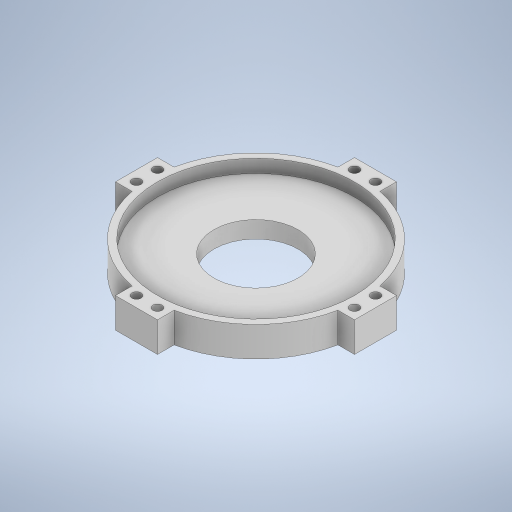
# Autodesk Inventor part: CO-0-01-PlanetaryCap
Saved by Autodesk Inventor 2023 (Build 270158000, 158)
## iProperties
Created: 2023-09-29
Part Number: CO-0-01-PlanetaryCap
Material: Generic
Document SubType Name: Modeling
Designer: thesl
Density: 1 g/cm^3
Appearance: Default
Author: thesl
Autodesk Inventor part; units mm, degrees
ref_plane "YZ Plane" through (0, 0, 0) normal (1, 0, 0) x (0, 1, 0)
ref_plane "XZ Plane" through (0, 0, 0) normal (0, 1, 0) x (-1, 0, 0)
ref_plane "XY Plane" through (0, 0, 0) normal (0, 0, 1) x (1, 0, 0)
sketch "Sketch1" plane through (0, 0, 0) normal (0, 1, 0) x (-1, 0, 0)
  circle A0 centre (0, 0) radius 50.8
  circle A1 centre (0, 0) radius 20.32
  dimension "d0" = 101.6
  dimension "d1" = 40.64
  constraints: 2 centre point, 2 coincident
  measures "d0" diameter of A0
  measures "d1" diameter of A1
extrude "Extrusion1" add sketch "Sketch1" along normal blind 14.5034
sketch "Sketch2" plane through (0, 14.5034, 0) normal (0, 1, 0) x (1, 0, 0)
  circle A0 centre (0, 0) radius 47.625
  dimension "d4" = 95.25
  constraints: 1 centre point, 1 coincident
  measures "d4" diameter of A0
extrude "Extrusion2" cut sketch "Sketch2" against normal blind 6.35
sketch "Sketch3" plane through (0, 14.5034, 0) normal (0, 1, 0) x (1, 0, 0)
  circle A0 centre (0, 0) radius 47.625 projected
  line L0 (-47.625, 0) -> (-57.785, 0)
  line L1 (-57.785, 0) -> (-57.785, 10.16)
  line L2 (-57.785, 10.16) -> (-47.625, 10.16)
  line L3 (-47.625, 10.16) -> (-47.625, -10.16)
  line L4 (-47.625, -10.16) -> (-57.785, -10.16)
  line L5 (-57.785, -10.16) -> (-57.785, 0)
  line L6 (0, 47.625) -> (0, 57.785)
  line L7 (0, 57.785) -> (10.16, 57.785)
  line L8 (10.16, 57.785) -> (10.16, 47.625)
  line L9 (10.16, 47.625) -> (-10.16, 47.625)
  line L10 (-10.16, 47.625) -> (-10.16, 57.785)
  line L11 (-10.16, 57.785) -> (0, 57.785)
  line L12 (47.625, 0) -> (57.785, 0)
  line L13 (57.785, 0) -> (57.785, 10.16)
  line L14 (57.785, 10.16) -> (47.625, 10.16)
  line L15 (47.625, 10.16) -> (47.625, -10.16)
  line L16 (47.625, -10.16) -> (57.785, -10.16)
  line L17 (57.785, -10.16) -> (57.785, 0)
  line L18 (0, -47.625) -> (0, -57.785)
  line L19 (0, -57.785) -> (10.16, -57.785)
  line L20 (10.16, -57.785) -> (10.16, -47.625)
  line L21 (10.16, -47.625) -> (-10.16, -47.625)
  line L22 (-10.16, -47.625) -> (-10.16, -57.785)
  line L23 (-10.16, -57.785) -> (0, -57.785)
  dimension "d7" = 10.16
  dimension "d8" = 10.16
  dimension "d9" = 20.32
  dimension "d10" = 10.16
  dimension "d11" = 10.16
  dimension "d12" = 10.16
  dimension "d13" = 20.32
  dimension "d14" = 10.16
  dimension "d15" = 10.16
  dimension "d16" = 10.16
  dimension "d17" = 20.32
  dimension "d18" = 10.16
  dimension "d19" = 10.16
  dimension "d20" = 10.16
  dimension "d21" = 10.16
  dimension "d22" = 20.32
  dimension "d23" = 10.16
  constraints: 48 end point, 10 perpendicular, 9 point on line, 4 point on circle, 3 parallel, 2 horizontal
  measures "d7" distance of L0.start L0.end
  measures "d8" distance of L0.end L1.end
  measures "d9" distance of L2.end L3.end
  measures "d10" distance of L6.start L6.end
  measures "d11" distance of L6.end L7.end
  measures "d12" distance of L7.end L8.end
  measures "d13" distance of L8.end L9.end
  measures "d14" distance of L9.end L10.end
  measures "d15" distance of L12.start L12.end
  measures "d16" distance of L12.end L13.end
  measures "d17" distance of L14.end L15.end
  measures "d18" distance of L15.end L16.end
  measures "d19" distance of L18.start L18.end
  measures "d20" distance of L18.end L19.end
  measures "d21" distance of L19.end L20.end
  measures "d22" distance of L20.end L21.end
  measures "d23" distance of L21.end L22.end
extrude "Extrusion3" add sketch "Sketch3" against normal up to surface (14.5034 mm away) contours L21 L20 L19 L18 | L18 L23 L22 L21 | L3 L4 L5 L0 | L0 L1 L2 L3 | L9 L10 L11 L6 | L6 L7 L8 L9 | L15 L14 L13 L12 | L12 L17 L16 L15
sketch "Sketch4" plane through (0, 14.5034, 0) normal (0, 1, 0) x (1, 0, 0)
  line L0 (-57.785, 10.16) -> (-57.785, -10.16) projected
  line L1 (-57.785, 10.16) -> (-52.705, 10.16)
  line L2 (-49.7736, 10.16) -> (-57.785, 10.16) projected
  line L3 (-52.705, 10.16) -> (-52.705, 5.08)
  line L4 (-52.705, 5.08) -> (-52.705, -5.08)
  line L5 (-10.16, 57.785) -> (-10.16, 49.7736) projected
  line L6 (-10.16, 57.785) -> (-10.16, 52.705)
  line L7 (-10.16, 52.705) -> (-5.08, 52.705)
  line L8 (-5.08, 52.705) -> (5.08, 52.705)
  line L9 (49.7736, 10.16) -> (57.785, 10.16) projected
  line L10 (57.785, 10.16) -> (52.705, 10.16)
  line L11 (52.705, 10.16) -> (52.705, 5.08)
  line L12 (52.705, 5.08) -> (52.705, -5.08)
  line L13 (10.16, -49.7736) -> (10.16, -57.785) projected
  line L14 (10.16, -57.785) -> (10.16, -52.705)
  line L15 (10.16, -52.705) -> (5.08, -52.705)
  line L16 (5.08, -52.705) -> (-5.08, -52.705)
  circle A0 centre (-52.705, -5.08) radius 2.2479
  circle A1 centre (-52.705, 5.08) radius 2.2479
  circle A2 centre (-5.08, 52.705) radius 2.2479
  circle A3 centre (5.08, 52.705) radius 2.2479
  circle A4 centre (52.705, 5.08) radius 2.2479
  circle A5 centre (52.705, -5.08) radius 2.2479
  circle A6 centre (-5.08, -52.705) radius 2.2479
  circle A7 centre (5.08, -52.705) radius 2.2479
  point P0 (0, 0)
  dimension "d26" = 5.08
  dimension "d27" = 5.08
  dimension "d28" = 10.16
  dimension "d29" = 5.08
  dimension "d30" = 5.08
  dimension "d31" = 10.16
  dimension "d32" = 5.08
  dimension "d33" = 5.08
  dimension "d34" = 10.16
  dimension "d35" = 5.08
  dimension "d36" = 5.08
  dimension "d37" = 10.16
  dimension "d38" = 4.4958
  dimension "d39" = 4.4958
  dimension "d40" = 4.4958
  dimension "d41" = 4.4958
  dimension "d42" = 4.4958
  dimension "d43" = 4.4958
  dimension "d44" = 4.4958
  constraints: 24 end point, 8 centre point, 8 coincident, 8 point on line, 4 perpendicular
  measures "d26" distance of L0.start L1.end
  measures "d27" distance of L1.end L3.end
  measures "d28" distance of L3.end L4.end
  measures "d29" distance of L5.start L6.end
  measures "d30" distance of L6.end L7.end
  measures "d31" distance of L7.end L8.end
  measures "d32" distance of L9.end L10.end
  measures "d33" distance of L10.end L11.end
  measures "d34" distance of L11.end L12.end
  measures "d35" distance of L13.end L14.end
  measures "d36" distance of L14.end L15.end
  measures "d37" distance of L15.end L16.end
  measures "d38" diameter of A0
  measures "d39" diameter of A2
  measures "d40" diameter of A3
  measures "d41" diameter of A4
  measures "d42" diameter of A5
  measures "d43" diameter of A6
  measures "d44" diameter of A7
extrude "Extrusion4" cut sketch "Sketch4" against normal blind 25.4
body "Solid1"
